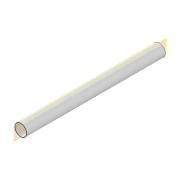
# Autodesk Inventor part: SlipersLåda 211018005
Saved by Autodesk Inventor 2020 (Build 240168000, 168)
## iProperties
Created: 2021-10-19
Part Number: SlipersLåda 211018005
Material: Generic
Document SubType Name: Modeling
Designer: dicpet001
Density: 1 g/cm^3
Appearance: Default
Author: dicpet001
Autodesk Inventor part; units mm, degrees
ref_plane "YZ Plane" through (0, 0, 0) normal (1, 0, 0) x (0, 1, 0)
ref_plane "XZ Plane" through (0, 0, 0) normal (0, 1, 0) x (-1, 0, 0)
ref_plane "XY Plane" through (0, 0, 0) normal (0, 0, 1) x (1, 0, 0)
sketch "Sketch1" plane through (0, 0, 0) normal (0, 0, 1) x (1, 0, 0)
  line L0 (0, 31.5) -> (0, -31.5) projected
  line L1 (-31.5, 0) -> (31.5, 0) projected
  circle A0 centre (0, 0) radius 22.5
  circle A1 centre (0, 0) radius 20.5
  dimension "d0" = 45
  dimension "d1" = 2
  dimension "d2" = 41
  constraints: 2 centre point, 1 coincident
  measures "d0" diameter of A0
  measures "d1" radial gap between concentric circles of A0 A1
  measures "d2" diameter of A1
extrude "Extrusion1" add sketch "Sketch1" against normal blind 510 contours A0 L1 A1 L0 | L0 A1 L1 A0 | A0 L0 A1 L1 | L1 A1 L0 A0
body "Solid1"
